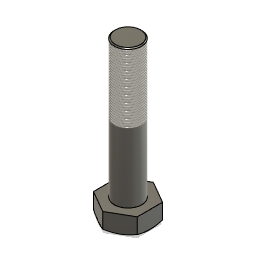
6432106821_ASM_10 (Autodesk Fusion 360 archive; units mm, degrees)
design "Hexagonal head bolt M12x1, 60 long, 30 thread length"
Autodesk Fusion 360 part; units mm, degrees
sketch "Sketch1" plane through (0, 0, 0) normal (0, 1, 0) x (1, 0, 0)
  line L0 (9.5, 5.4848) -> (0, 10.9697)
  line L1 (0, 10.9697) -> (-9.5, 5.4848)
  line L2 (-9.5, 5.4848) -> (-9.5, -5.4848)
  line L3 (-9.5, -5.4848) -> (0, -10.9697)
  line L4 (0, -10.9697) -> (9.5, -5.4848)
  line L5 (9.5, -5.4848) -> (9.5, 5.4848)
  dimension "d1" = 9.5
  measures "d1" distance of origin L5
extrude "Extrude1" add sketch "Sketch1" along normal blind 7.5
sketch "Sketch2" plane through (0, 7.5, 0) normal (0, 1, 0) x (-1, 0, 0)
  line L0 (-9.5, 5.4848) -> (-9.5, -5.4848)
  line L1 (-9.5, -5.4848) -> (0, -10.9697)
  line L2 (0, -10.9697) -> (9.5, -5.4848)
  line L3 (9.5, -5.4848) -> (9.5, 5.4848)
  line L4 (9.5, 5.4848) -> (0, 10.9697)
  line L5 (0, 10.9697) -> (-9.5, 5.4848)
  circle A0 centre (0, 0) radius 6
  dimension "d4" = 12
  constraint coincident A0.centre origin
  measures "d4" diameter of A0
extrude "Extrude2" add sketch "Sketch2" along normal blind 60 contours A0
thread "Thread1" "ISO Metric profile 12.0 M12x1 6g" major diameter 11.884 minor diameter 10.7405 pitch 1 angle 60 resizes the face on face at (-5.9702, 47.5, -0.5974) from (0, 37.5, 0) to (0, 67.5, 0)
sketch "Sketch3" plane through (0, 0, 0) normal (0, -1, 0) x (1, 0, 0)
  line L0 (9.5, -5.4848) -> (9.5, 5.4848)
  line L1 (9.5, 5.4848) -> (0, 10.9697)
  line L2 (0, 10.9697) -> (-9.5, 5.4848)
  line L3 (-9.5, 5.4848) -> (-9.5, -5.4848)
  line L4 (-9.5, -5.4848) -> (0, -10.9697)
  line L5 (0, -10.9697) -> (9.5, -5.4848)
  circle A0 centre (0, 0) radius 9.5
  line L6 (0, 10.9697) -> (0, 9.5)
  constraint coincident A0.centre origin
  constraint tangent L0 A0
  constraint coincident L1.end L2.start
  constraint coincident A0 L6.end
  constraint vertical L6
sketch "Sketch5" plane through (0, 0, 0) normal (1, 0, 0) x (0, 0, -1)
  line L0 (-10.9697, 0.8487) -> (-9.4997, 0)
  line L1 (-10.9697, 0) -> (-10.9697, 7.5)
  line L2 (-9.5, 0) -> (9.5, 0)
  line L3 (-10.9697, 0) -> (-9.5, 0)
  point P0 (-10.9697, 0)
  dimension "d9" = 1.47
  dimension "d10" = 30
  constraint coincident L0.start L1
  constraint coincident L0.end L2
  measures "d9" distance of L0.end P0
  measures "d10" angle of L0 L3
revolve "Revolve1" cut sketch "Sketch5" angle 360 about axis through (0, 1.75, 0) along (0, 1, 0)
sketch "Sketch6" plane through (0, 0, 0) normal (0, 0, 1) x (1, 0, 0)
  line L0 (-6, 67.5) -> (-6, 67)
  line L1 (-6, 67) -> (-5.5, 67.5)
  line L2 (-5.5, 67.5) -> (-6, 67.5)
  dimension "d12" = 0.5
  dimension "d13" = 45
  constraint vertical L0
  measures "d12" distance of L0.start L0.end
  measures "d13" angle of L0 L1
revolve "Revolve2" cut sketch "Sketch6" angle 360 about axis through (0, 1.75, 0) along (0, 1, 0)
equation "d1 = ( 19 / 2 ) * 1 mm"
